HDPE test circle 2 mm cutter 12point8 circle centered 3point8 height_v1 (Autodesk Fusion 360 design; units mm, degrees)
Autodesk Fusion 360 part; units mm, degrees
sketch "movingPlatform" plane through (0, 0, 0) normal (0, 0, 1) x (1, 0, 0)
  circle A0 centre (0, 0) radius 6.4
  line L0 (6.4, -6.4) -> (-6.4, -6.4)
  line L1 (-6.4, -6.4) -> (-6.4, 6.4)
  line L2 (-6.4, 6.4) -> (6.4, 6.4)
  line L3 (6.4, 6.4) -> (6.4, -6.4)
  line L4 (6.4, -6.4) -> (-6.4, 6.4) construction
  line L5 (-6.4, -6.4) -> (6.4, 6.4) construction
  dimension "d65" = 12.8
  dimension "d81" = 12.8
  dimension "d82" = 12.8
  constraint coincident A0.centre origin
  constraint horizontal L0
  constraint perpendicular L0 L1
  constraint parallel L0 L2
  constraint parallel L1 L3
  constraint coincident L4 A0.centre
  constraint coincident L5 A0.centre
  measures "d65" diameter of A0
  measures "d81" distance of L0.start L0.end
  measures "d82" distance of L0.start L2.end
extrude "Extrude16" add sketch "movingPlatform" along normal blind 3.8 contours A0 L0 L3 | A0 L2 L3 | A0 L1 L2 | A0 L0 L1
